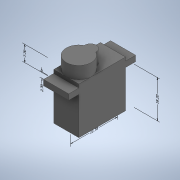
# Autodesk Inventor part: Servo
Saved by Autodesk Inventor 2020.4 (Build 244396000, 396)
## iProperties
Created: 2021-02-03
Part Number: Servo
Material: Generic
Document SubType Name: Modeling
Designer: armin
Density: 1 g/cm^3
Appearance: Default
Author: armin
Autodesk Inventor part; units mm, degrees
ref_plane "YZ Plane" through (0, 0, 0) normal (1, 0, 0) x (0, 1, 0)
ref_plane "XZ Plane" through (0, 0, 0) normal (0, 1, 0) x (-1, 0, 0)
ref_plane "XY Plane" through (0, 0, 0) normal (0, 0, 1) x (1, 0, 0)
sketch "Sketch1" plane through (0, 0, 0) normal (0, 1, 0) x (-1, 0, 0)
  line L0 (0, 0) -> (12.2, 0)
  line L1 (12.2, 0) -> (12.2, -22.7)
  line L2 (12.2, -22.7) -> (0, -22.7)
  line L3 (0, -22.7) -> (0, 0)
  dimension "d0" = 12.2
  dimension "d1" = 22.7
  constraints: 8 end point, 2 parallel, 1 horizontal, 1 perpendicular
  measures "d0" distance of L1.end L2.end
  measures "d1" distance of L0.end L1.end
extrude "Extrusion1" add sketch "Sketch1" along normal blind 18.2
sketch "Sketch2" plane through (0, 18.2, 0) normal (0, 1, 0) x (1, 0, 0)
  line L0 (-12.2, -4.9) -> (0, -4.9)
  line L1 (0, -4.9) -> (0, 27.6)
  line L2 (0, 27.6) -> (-12.2, 27.6)
  line L3 (-12.2, 27.6) -> (-12.2, -4.9)
  line L4 (-12.2, -4.9) -> (0, 27.6) construction
  line L5 (0, -4.9) -> (-12.2, 27.6) construction
  line L6 (-12.2, 0) -> (0, 0) projected
  line L7 (-12.2, 22.7) -> (-12.2, 0) projected
  point P0 (-6.1, 11.35)
  dimension "d4" = 32.5
  dimension "d5" = 12.2
  dimension "d6" = 11.35
  dimension "d7" = 6.1
  constraints: 12 end point, 2 midpoint, 2 parallel, 1 horizontal, 1 perpendicular
  measures "d4" distance of L1.end L0.end
  measures "d5" distance of L0.start L0.end
  measures "d6" distance from line of point (-6.1, 11.35) L6
  measures "d7" distance from line of point (-6.1, 11.35) L7
extrude "Extrusion2" add sketch "Sketch2" along normal blind 2.7
sketch "Sketch3" plane through (0, 20.9, 0) normal (0, 1, 0) x (1, 0, 0)
  line L0 (0, 22.7) -> (-12.2, 22.7) projected
  line L1 (0, 0) -> (-12.2, 0)
  line L2 (-12.2, 0) -> (-12.2, 22.7)
  line L3 (-12.2, 22.7) -> (0, 22.7)
  line L4 (0, 22.7) -> (0, 0)
  constraints: 8 end point, 2 parallel, 1 horizontal, 1 perpendicular
extrude "Extrusion3" add sketch "Sketch3" along normal blind 1.7
sketch "Sketch5" plane through (0, 22.6, 0) normal (0, 1, 0) x (1, 0, 0)
  circle A0 centre (-6.1, 6.1) radius 6.1
  line L0 (-12.2, 22.7) -> (-12.2, 0) projected
  line L1 (0, 0) -> (0, 22.7) projected
  line L2 (-12.2, 0) -> (0, 0) projected
  circle A1 centre (-6.1, 11.8) radius 2.8
  point P0 (-8.8866, 11.5263)
  point P1 (-3.3134, 11.5263)
  dimension "d12" = 6.1
  dimension "d13" = 5.6
  dimension "d14" = 14.6
  constraints: 2 centre point, 2 tangent
  measures "d12" distance from line of L1 A0.centre
  measures "d13" diameter of A1
extrude "Extrusion4" add sketch "Sketch5" along normal blind 6 contours A0 A1 | A1 A0 | A0 A1
fillet "Fillet1" radius 0.25 2 edges at (-8.8866, 25.6, -11.5263) (-3.3134, 25.6, -11.5263)
body "Solid1"
